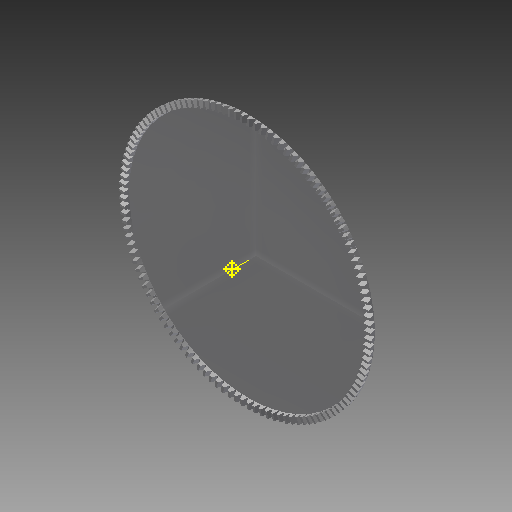
# Autodesk Inventor part: Bevel Gear1
Saved by Autodesk Inventor 2017 (Build 210142000, 142)
## iProperties
Created: 2017-01-10
Part Number: Bevel Gear1
Material: Steel, Mild
Document SubType Name: Modeling
Designer: David Kopala
Categories: <?xml version="1.0" encoding="UTF-16"?> <MemberInstance><Categories><FamilyTemplate><FamilyTemplateParameter ValueType="xs:double" Id="1" ObjectReferenceKey="da_z" ObjectType="kUserParameterObject"/><FamilyTemplateParameter ValueType="xs:double" Id="2" ObjectReferenceKey="da_b" ObjectType="kUserParameterObject"/><FamilyTemplateParameter ValueType="xs:double" Id="3" ObjectReferenceKey="da_beta" ObjectType="kUserParameterObject"/><FamilyTemplateParameter ValueType="xs:double" Id="4" ObjectReferenceKey="da_dae" ObjectType="kUserParameterObject"/><FamilyTemplateParameter ValueType="xs:double" Id="5" ObjectReferenceKey="da_ve" ObjectType="kUserParameterObject"/><FamilyTemplateParameter ValueType="xs:double" Id="6" ObjectReferenceKey="da_omega" ObjectType="kUserParameterObject"/><FamilyTemplateParameter ValueType="xs:string" Id="7" ObjectReferenceKey="EAIAABAAAAAAHwAAAAAAAIAAAAAAAAAA" ObjectType="83914240" SubObjectId="SurfaceGeometry"/></FamilyTemplate><ParamToTemplateMap><ParamToTemplate CategoryParameter="//CategoryParameter[@InternalName='046C89C9-8512-4d59-83FE-43B91F4F132A']" TemplateParameter="1"/><ParamToTemplate CategoryParameter="//CategoryParameter[@InternalName='2552DF32-E462-4b46-AEBF-C6C7768E72AC']" TemplateParameter="2"/><ParamToTemplate CategoryParameter="//CategoryParameter[@InternalName='C9EE641D-15FC-4fae-A226-E94C4372FDD7']" TemplateParameter="3"/><ParamToTemplate><ParamToTemplate CategoryParameter="//CategoryParameter[@InternalName='00B6519A-459B-49c7-AD84-2E56D39A5744']" ConstantValue="0.000000"/></ParamToTemplate><ParamToTemplate><ParamToTemplate CategoryParameter="//CategoryParameter[@InternalName='04B31F0E-C7A6-4894-AA32-9629BEFACF47']" ConstantValue="1.000000"/></ParamToTemplate><ParamToTemplate><ParamToTemplate CategoryParameter="//CategoryParameter[@InternalName='43CBEC2E-7847-49e7-A936-2F7889FCB2D9']" ConstantValue="0.200000"/></ParamToTemplate><ParamToTemplate><ParamToTemplate CategoryParameter="//CategoryParameter[@InternalName='B1EFC894-105D-4ebd-86BF-FA20ED196853']" ConstantValue="0.300000"/></ParamToTemplate><ParamToTemplate><ParamToTemplate CategoryParameter="//CategoryParameter[@InternalName='51175063-3D10-4879-93E8-6246FE8B403D']" ConstantValue="2061532430.657340"/></ParamToTemplate><ParamToTemplate><ParamToTemplate CategoryParameter="//CategoryParameter[@InternalName='A3A52E27-4454-46a9-B0BD-C932399B70AF']" ConstantValue="0.300000"/></ParamToTemplate><ParamToTemplate CategoryParameter="//CategoryParameter[@InternalName='2A200944-5A8C-41ca-B96E-8520D2E510F1']" TemplateParameter="4"/><ParamToTemplate><ParamToTemplate CategoryParameter="//CategoryParameter[@InternalName='1A637F62-92C8-44bc-B81F-10802510B579']" ConstantValue="29.534356"/></ParamToTemplate><ParamToTemplate CategoryParameter="//CategoryParameter[@InternalName='B52DD4BE-6863-48fb-BF58-89EF6F9EC65C']" TemplateParameter="5"/><ParamToTemplate><ParamToTemplate CategoryParameter="//CategoryParameter[@InternalName='3956BFF2-84D2-457d-93C2-9B0613DEBA67']" ConstantValue="1.572216"/></ParamToTemplate><ParamToTemplate CategoryParameter="//CategoryParameter[@InternalName='739CFA02-461B-4bf8-8049-181FCAD8B28F']" TemplateParameter="6"/><ParamToTemplate><ParamToTemplate CategoryParameter="//CategoryParameter[@InternalName='A27E999F-E2CE-4481-8A2A-EBF499C4C3C5']" ConstantValue="0.000000"/></ParamToTemplate><ParamToTemplate><ParamToTemplate CategoryParameter="//CategoryParameter[@InternalName='9E1B4470-B2D3-4ff1-B813-535BB4CDF51A']" ConstantValue="3523220.976809"/></ParamToTemplate><ParamToTemplate><ParamToTemplate CategoryParameter="//CategoryParameter[@InternalName='F8452263-BFF6-458c-9FB1-07C4B99E95CD']" ConstantValue="11397033.805607"/></ParamToTemplate><ParamToTemplate><ParamToTemplate CategoryParameter="//CategoryParameter[@InternalName='3E3BB259-FD49-497f-8171-6EBC954A3479']" ConstantValue="2.000000"/></ParamToTemplate><ParamToTemplate CategoryParameter="//CategoryParameter[@InternalName='27C3BAF2-7550-4e4b-AE2C-0DB134B7D9B7']" TemplateParameter="7"/></ParamToTemplateMap><Category DisplayName="Gear" InternalName="DC85795E-93AB-48d5-8EEE-5A27447B64BD" Mnemonic="Gear"><CategoryParameter DisplayName="z" InternalName="046C89C9-8512-4d59-83FE-43B91F4F132A" Mnemonic="z"/><CategoryParameter DisplayName="b" InternalName="2552DF32-E462-4b46-AEBF-C6C7768E72AC" Mnemonic="b"/><CategoryParameter DisplayName="||b|" InternalName="C9EE641D-15FC-4fae-A226-E94C4372FDD7" Mnemonic="beta"/><CategoryParameter DisplayName="x" InternalName="00B6519A-459B-49c7-AD84-2E56D39A5744" Mnemonic="x"/><CategoryParameter DisplayName="a*" InternalName="04B31F0E-C7A6-4894-AA32-9629BEFACF47" Mnemonic="a"/><CategoryParameter DisplayName="c*" InternalName="43CBEC2E-7847-49e7-A936-2F7889FCB2D9" Mnemonic="c"/><CategoryParameter DisplayName="r|.f|*" InternalName="B1EFC894-105D-4ebd-86BF-FA20ED196853" Mnemonic="rf"/><CategoryParameter DisplayName="E" InternalName="51175063-3D10-4879-93E8-6246FE8B403D" Mnemonic="E"/><CategoryParameter DisplayName="||m|" InternalName="A3A52E27-4454-46a9-B0BD-C932399B70AF" Mnemonic="mi"/><Category DisplayName="BevelGear" InternalName="0C98F69A-0C2B-4791-B2FE-7691BB227E77" Mnemonic="BevelGear"><CategoryParameter DisplayName="d|.ae|" InternalName="2A200944-5A8C-41ca-B96E-8520D2E510F1" Mnemonic="dae"/><CategoryParameter DisplayName="d|.ai|" InternalName="1A637F62-92C8-44bc-B81F-10802510B579" Mnemonic="dai"/><CategoryParameter DisplayName="A|.e|" InternalName="B52DD4BE-6863-48fb-BF58-89EF6F9EC65C" Mnemonic="ve"/><CategoryParameter DisplayName="A|.i|" InternalName="3956BFF2-84D2-457d-93C2-9B0613DEBA67" Mnemonic="vi"/><CategoryParameter DisplayName="||S|" InternalName="739CFA02-461B-4bf8-8049-181FCAD8B28F" Mnemonic="omega"/><CategoryParameter DisplayName="x|.t|" InternalName="A27E999F-E2CE-4481-8A2A-EBF499C4C3C5" Mnemonic="xt"/><CategoryParameter DisplayName="||s||.Flim|" InternalName="9E1B4470-B2D3-4ff1-B813-535BB4CDF51A" Mnemonic="sFlim"/><CategoryParameter DisplayName="||s||.Hlim|" InternalName="F8452263-BFF6-458c-9FB1-07C4B99E95CD" Mnemonic="sHlim"/><CategoryParameter DisplayName="type" InternalName="3E3BB259-FD49-497f-8171-6EBC954A3479" Mnemonic="type"/><CategoryParameter DisplayName="PitchDiameter" InternalName="27C3BAF2-7550-4e4b-AE2C-0DB134B7D9B7" Mnemonic="IDS_PITCHDIAM"/></Category></Category></Categories></MemberInstance>
Mass: 60.9118 g
Surface Area: 34.3074 cm^2
Volume: 7.7496 cm^3
Density: 7.86 g/cm^3
Appearance: Steel
CustomPartVersion: 1
Author: David Kopala
Autodesk Inventor part; units mm, degrees
ref_plane "XZ Plane" through (0, 0, 0) normal (0, 1, 0) x (-1, 0, 0)
ref_plane "Mesh Plane2" through (0, 0, 0) normal (0.9996685, 0.0257479, 0) x (0, 0, 1)
sketch "Teeth Body Sketch" plane through (0, 0, 0) normal (1, 0, 0) x (0, 1, 0)
  line L0 (0, 0) -> (154.568, -22.0752) construction
  line L1 (154.568, -22.0752) -> (155.25, -16.529)
  line L2 (155.25, -16.529) -> (0, 0) construction
  line L3 (154.94, -19.05) -> (0, 0) construction
  line L4 (147.0232, -20.9977) -> (147.6718, -15.7222)
  line L5 (154.568, -22.0752) -> (147.0232, -20.9977)
  line L6 (155.25, -16.529) -> (147.6718, -15.7222)
  line L7 (0, -26.4907) -> (0, 4.4151) projected
  line L8 (0, -19.05) -> (155.25, -19.05) construction
  dimension "d0" = 309.88
  dimension "d1" = 309.1361
  dimension "d2" = 310.4999
  dimension "d3" = 7.62
  dimension "d4" = 16.529
  constraints: 16 end point, 4 point on line, 3 perpendicular, 2 collinear, 1 horizontal alignment, 1 vertical alignment
  measures "d0" diameter of L3.start L7
  measures "d1" diameter of L0.end L7
  measures "d2" diameter of L1.end L7
  measures "d3" distance between parallel lines of L1 L4
  measures "d4" vertical distance of L1.end L0.start
revolve "Teeth Body" add sketch "Teeth Body Sketch" angle 360 about axis through (0, 0, 0) along (0, 0, 1)
ref_plane "Tooth Plane" through (0, 154.94, -19.05) normal (0, -0.9925262, 0.1220319) x (1, 0, 0)
sketch "Start Sketch" plane through (0, 154.94, -19.05) normal (0, -0.9925262, 0.1220319) x (1, 0, 0)
  line L0 (0, -1549.3378) -> (0, 263.1443) projected
  arc A0 (-0.7245, -3.7186) -> (-3.4804, 4.2116) centre (-413.1132, -142.5872) ccw
  arc A1 (3.4804, 4.2116) -> (0.7245, -3.7186) centre (413.1132, -142.5872) ccw
  line L1 (-0.7245, -3.7186) -> (0.7245, -3.7186)
  arc A2 (3.4804, 4.2116) -> (-3.4804, 4.2116) centre (0, -1269.668) ccw
  dimension "d7" = 435.1424
  dimension "d8" = 413.1132
  dimension "d9" = 1127.0807
  dimension "d57" = 1273.8843
  dimension "d58" = 1265.9494
  constraints: 6 point on circle, 3 centre point, 3 symmetric about line, 2 end point, 1 coincident, 1 perpendicular, 1 other
  measures "d7" radius of A0
  measures "d8" horizontal distance of point (0, -1269.668) A0.centre
  measures "d9" vertical distance of point (0, -1269.668) A0.centre
  measures "d57" radius of A2
  measures "d58" distance from line of A2.centre L1
sketch "End Sketch" plane through (0, 147.0996, -18.086) normal (0, -0.9925262, 0.1220319) x (1, 0, 0)
  line L0 (0, -1471.8243) -> (0, 251.4888) projected
  arc A0 (-0.6886, -2.2645) -> (-3.3078, 5.2724) centre (-392.6217, -134.2449) ccw
  arc A1 (3.3078, 5.2724) -> (0.6886, -2.2645) centre (392.6217, -134.2449) ccw
  line L1 (-0.6886, -2.2645) -> (0.6886, -2.2645)
  arc A2 (3.3078, 5.2724) -> (-3.3078, 5.2724) centre (0, -1205.4195) ccw
  dimension "d12" = 413.5582
  dimension "d15" = 392.6217
  dimension "d16" = 1071.1746
  dimension "d59" = 1210.6964
  dimension "d60" = 1203.155
  constraints: 6 point on circle, 3 centre point, 3 symmetric about line, 2 end point, 1 coincident, 1 other
  measures "d12" radius of A0
  measures "d15" horizontal distance of A0.centre point (0, -1205.419)
  measures "d16" vertical distance of A0.centre point (0, -1205.419)
  measures "d59" radius of A2
  measures "d60" distance from line of A2.centre L1
loft "Loft" cut profiles "Start Sketch", "End Sketch"
pattern_circular "Circular Pattern" count 122 over 360 about axis through (0, 0, 0) along (0, 0, 1) of "Loft"
ref_plane "End Plane" through (0, 147.0996, -18.086) normal (0, -0.9925262, 0.1220319) x (1, 0, 0)
sketch3d "3D Sketch Right"
ref_plane "End Plane Right" through (-2.8354, 147.0723, -18.086) normal (0.0191313, -0.9923418, 0.1220319) x (0.9998142, 0.0192754, 0)
sketch "End Sketch Right" plane through (-2.8354, 147.0723, -18.086) normal (0.0191313, -0.9923418, 0.1220319) x (0.9998142, 0.0192754, 0)
  arc A0 (-0.6886, -2.2645) -> (-3.3078, 5.2724) centre (-392.6217, -134.2449) ccw
  line L0 (0, -1474.4528) -> (0, 254.1173) projected
  arc A1 (3.3078, 5.2724) -> (0.6886, -2.2645) centre (392.6217, -134.2449) ccw
  line L1 (-0.6886, -2.2645) -> (0.6886, -2.2645)
  arc A2 (3.3078, 5.2724) -> (-3.3078, 5.2724) centre (0, -1205.4195) ccw
  dimension "d70" = 392.6217
  dimension "d71" = 1071.1746
  dimension "d72" = 413.5582
  dimension "d73" = 1203.155
  dimension "d74" = 1210.6964
  constraints: 6 point on circle, 3 centre point, 3 symmetric about line, 2 end point, 1 coincident, 1 perpendicular, 1 other
  measures "d70" horizontal distance of A2.centre A0.centre
  measures "d71" vertical distance of point (0, -1205.419) A0.centre
  measures "d72" radius of A0
  measures "d73" distance from line of point (0, -1205.419) L1
  measures "d74" radius of A2
feature "Loft Right" [suppressed]
pattern_circular "Circular Pattern Right" [suppressed]
sketch3d "3D Sketch Left"
ref_plane "End Plane Left" through (2.8457, 147.0723, -18.1168) normal (-0.0192001, -0.9923153, 0.1222364) x (0.9998129, -0.0193452, 0)
sketch "End Sketch Left" plane through (2.8457, 147.0723, -18.1168) normal (-0.0192001, -0.9923153, 0.1222364) x (0.9998129, -0.0193452, 0)
  line L0 (0, -1474.4362) -> (0, 254.1618) projected
  arc A0 (-0.6886, -2.2339) -> (-3.3078, 5.3029) centre (-392.6217, -134.2143) ccw
  arc A1 (3.3078, 5.3029) -> (0.6886, -2.2339) centre (392.6217, -134.2143) ccw
  line L1 (-0.6886, -2.2339) -> (0.6886, -2.2339)
  ellipse E0 centre (0, -15.6043) end of major axis (147.6718, -15.6043) minor radius 18.0509 projected
  arc A2 (3.3078, 5.3029) -> (-3.3078, 5.3029) centre (0, -1205.3889) ccw
  dimension "d56" = 18.0509
  dimension "d30" = 413.5582
  dimension "d31" = 392.6217
  dimension "d32" = 1071.1746
  dimension "d61" = 1210.6964
  dimension "d62" = 1203.155
  constraints: 6 point on circle, 3 centre point, 3 symmetric about line, 2 end point, 1 coincident, 2 other
  measures "d30" radius of A0
  measures "d31" horizontal distance of point (0, -1205.389) A0.centre
  measures "d32" vertical distance of A0.centre point (0, -1205.389)
  measures "d61" radius of A2
  measures "d62" distance from line of point (0, -1205.389) L1
feature "Loft Left" [suppressed]
pattern_circular "Circular Pattern Left" [suppressed]
sketch "Body Sketch" plane through (0, 0, 0) normal (1, 0, 0) x (0, 1, 0)
  line L0 (0, -22.2894) -> (0, -20.7929) projected
  line L1 (154.568, -22.0752) -> (147.0232, -20.9977) projected
  line L2 (147.0232, -20.9977) -> (0, -20.9977)
  line L3 (154.568, -22.0752) -> (0, -22.0752)
  constraints: 4 end point, 2 perpendicular, 2 point on line
revolve "Fix Body" add sketch "Body Sketch" angle 360 about axis through (0, 0, 0) along (0, 0, 1)
sketch "Sketch6" plane through (0, 0, 0) normal (1, 0, 0) x (0, 1, 0)
  line L0 (154.94, -19.05) -> (0, 0) projected
  line L1 (0, -22.86) -> (0, 3.81) projected
surface revolve "Pitch Diameter" sketch "Sketch6" angle 360 about axis through (0, 0, 0) along (0, 0, 1) shown no curves L0
equation "\"d0\" = da_de"
equation "\"d1\" = da_dfe"
equation "\"d2\" = da_dae"
equation "\"d3\" = da_b"
equation "\"d4\" = da_ve"
equation "\"d7\" = fd_rr"
equation "\"d8\" = fd_x"
equation "\"d9\" = fd_y"
equation "\"d57\" = 0.5 * fd_dva + 0.3 * da_he"
equation "\"d58\" = 0.5 * fd_dva - 1.12 * da_he"
equation "\"da_teethtype\" = 0"
equation "\"da_b\" = 7.62"
equation "\"da_de\" = 309.88"
equation "\"da_dae\" = 310.49992"
equation "\"da_dfe\" = 309.13609"
equation "\"da_le\" = 156.10671"
equation "\"da_omega\" = 90deg"
equation "\"da_beta\" = 0"
equation "\"da_delta\" = 82.990616deg"
equation "\"da_alpha\" = 20deg"
equation "\"da_he\" = 5.588"
equation "\"da_ve\" = 16.52898"
equation "\"da_zv\" = 999.738535"
equation "\"fd_loft\" = da_b + 0.05 * da_he"
equation "\"fd_x\" = fd_x1 + fd_x2"
equation "\"fd_y\" = fd_y1 - fd_y2"
equation "\"fd_dd\" = fd_dva - 0.8 * da_he"
equation "\"da_dvw\" = 2539.33588"
equation "\"d11\" = fd_loft"
equation "\"da_dm\" = 302.31695"
equation "\"da_x\" = 0"
equation "\"da_m\" = 2.54"
equation "\"d50\" = da_omega"
equation "\"fd_rr\" = 435.14238"
equation "\"fd_dva\" = 2544.415877"
equation "\"fd_x1\" = 1.994911"
equation "\"fd_x2\" = 411.118257"
equation "\"fd_y1\" = 1269.666372"
equation "\"fd_y2\" = 142.585657"
body "Solid1"
body "Srf1"
